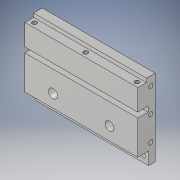
# Autodesk Inventor part: Стенка толстая
Saved by Autodesk Inventor 2019 (Build 230136000, 136)
## iProperties
Company: КВ33
Created: 2021-03-13
Part Number: Стенка толстая
Material: Типовые
Document SubType Name: Modeling
Designer: Петров Иван
Density: 1 g/cm^3
Appearance: Aluminum - Polished
Author: Петров Иван
Autodesk Inventor part; units mm, degrees
ref_plane "YZ Plane" through (0, 0, 0) normal (1, 0, 0) x (0, 1, 0)
ref_plane "XZ Plane" through (0, 0, 0) normal (0, 1, 0) x (-1, 0, 0)
ref_plane "XY Plane" through (0, 0, 0) normal (0, 0, 1) x (1, 0, 0)
sketch "Sketch1" plane through (0, 0, 0) normal (0, 0, 1) x (1, 0, 0)
  line L0 (50.1275, 12.4589) -> (-37.8725, 12.4589) projected
  line L1 (50.1275, 12.4589) -> (-37.8725, 12.4589)
  line L2 (-37.8725, 12.4589) -> (-37.8725, 62.4589)
  line L3 (-37.8725, 62.4589) -> (50.1275, 62.4589)
  line L4 (50.1275, 62.4589) -> (50.1275, 12.4589)
  circle A0 centre (-33.8725, 7.4589) radius 1.75 projected
  circle A1 centre (-13.8725, 7.4589) radius 1.75 projected
  circle A2 centre (6.1275, 7.4589) radius 1.75 projected
  circle A3 centre (26.1275, 7.4589) radius 1.75 projected
  circle A4 centre (46.1275, 7.4589) radius 1.75 projected
  line L5 (-37.8725, 2.4589) -> (50.1275, 2.4589) projected
  line L6 (-37.8725, 2.4589) -> (-37.8725, 12.4589) projected
  line L7 (50.1275, 12.4589) -> (-37.8725, 12.4589) projected
  line L8 (50.1275, 2.4589) -> (50.1275, 12.4589) projected
  line L9 (50.1275, -7.5411) -> (-37.8725, -7.5411) projected
  line L10 (-37.8725, -7.5411) -> (-37.8725, 2.4589) projected
  line L11 (50.1275, 2.4589) -> (-37.8725, 2.4589) projected
  line L12 (50.1275, -7.5411) -> (50.1275, 2.4589) projected
  dimension "d0" = 50
  dimension "d1" = 88
  constraints: 8 end point, 2 parallel, 1 horizontal, 1 perpendicular
  measures "d0" distance of L1.end L2.end
  measures "d1" distance of L2.end L3.end
ref_plane "Work Plane1" through (-40.3725, -19.5411, 5) normal (0, 0, -1) x (0, 1, 0)
extrude "Extrusion1" add sketch "Sketch1" along normal up to surface (5 mm away) contours L8 L5 L6 L0
sketch "Sketch2" plane through (0, 0, 0) normal (0, 0, -1) x (-1, 0, 0)
  line L0 (37.8725, -7.5411) -> (-50.1275, -7.5411)
  line L1 (-50.1275, -7.5411) -> (-50.1275, 2.4589)
  line L2 (37.8725, 2.4589) -> (-50.1275, 2.4589)
  line L3 (37.8725, -7.5411) -> (37.8725, 2.4589)
  circle A0 centre (-46.1275, 7.4589) radius 1.75
  circle A1 centre (-26.1275, 7.4589) radius 1.75
  circle A2 centre (-6.1275, 7.4589) radius 1.75
  circle A3 centre (13.8725, 7.4589) radius 1.75
  circle A4 centre (33.8725, 7.4589) radius 1.75
  line L4 (-50.1275, 2.4589) -> (37.8725, 2.4589)
  line L5 (-50.1275, 2.4589) -> (-50.1275, 12.4589)
  line L6 (37.8725, 12.4589) -> (-50.1275, 12.4589)
  line L7 (37.8725, 2.4589) -> (37.8725, 12.4589)
  line L8 (37.8725, 12.4589) -> (-50.1275, 12.4589)
  line L9 (-50.1275, 12.4589) -> (-50.1275, 62.4589)
  line L10 (-50.1275, 62.4589) -> (37.8725, 62.4589)
  line L11 (37.8725, 62.4589) -> (37.8725, 12.4589)
  line L12 (-50.1275, 2.4589) -> (-50.1275, 12.4589) projected
  point P0 (0, 0)
  point P1 (-12.255, 0)
  dimension "d4" = 50
  dimension "d5" = 88
  constraints: 24 end point, 5 centre point, 2 parallel, 1 horizontal, 1 perpendicular
  measures "d4" distance of L8.end L9.end
  measures "d5" distance of L9.end L10.end
ref_plane "Work Plane2" through (-22.976, -19.3597, 13.5507) normal (0, 0, 1) x (1, 0, 0)
extrude "Extrusion2" add sketch "Sketch2" against normal up to surface (13.5507 mm away) contours L6 L9 L10 L11
sketch "Sketch6" plane through (-37.8725, 62.4589, 0) normal (0, 1, 0) x (1, 0, 0)
  line L0 (88, -13.5507) -> (0, -13.5507) projected
  line L1 (88, 0) -> (88, -13.5507) projected
  line L2 (0, -13.5507) -> (88, -13.5507)
  line L3 (88, -13.5507) -> (88, -6.7754)
  line L4 (88, -6.7754) -> (0, -6.7754)
  line L5 (0, -6.7754) -> (0, -13.5507)
  point P0 (37.8725, 0)
  constraints: 8 end point, 2 parallel, 1 horizontal, 1 midpoint, 1 perpendicular
extrude "Extrusion6" cut sketch "Sketch6" against normal blind 3
sketch "Sketch7" plane through (50.1275, 2.4589, 5) normal (1, 0, 0) x (0, 0, -1)
  circle A0 centre (1.6123, 52.8914) radius 1.75
  line L0 (5, 0) -> (5, 60) projected
  line L1 (-1.7754, 60) -> (-1.7754, 57) projected
  point P0 (5, -2.4589)
  dimension "d30" = 3.5
  dimension "d31" = 3.3877
  dimension "d32" = 6.7754
  constraints: 1 centre point
  measures "d30" diameter of A0
  measures "d31" distance from line of L0 A0.centre
  measures "d32" distance between parallel lines of L0 L1
hole "Hole1" at (50.1275, 55.3502, 3.3877) direction (-1, 0, 0) diameter 3.5 depth 10 tip angle 120
thread "Thread2" size "M3.5x0.6" class "6H" standard "ANSI Metric M Profile" full length
pattern_linear "Rectangular Pattern2" count 3 spacing 19 along (0, -1, 0) of "Hole1"
ref_plane "Work Plane5" through (6.1275, 62.4589, 0) normal (1, 0, 0) x (0, 0, -1)
mirror "Mirror2" about plane through (6.1275, 62.4589, 0) normal (1, 0, 0) of "Hole1", "Rectangular Pattern2"
sketch "Sketch8" plane through (-37.8725, 59.4589, 0) normal (0, 1, 0) x (1, 0, 0)
  circle A0 centre (84, -10.0507) radius 1.75
  line L0 (88, -13.5507) -> (0, -13.5507) projected
  line L1 (88, -6.7754) -> (88, -13.5507) projected
  point P0 (37.8725, 0)
  dimension "d45" = 3.5
  dimension "d46" = 3.5
  dimension "d47" = 4
  constraints: 1 centre point
  measures "d45" diameter of A0
  measures "d46" distance from line of L0 A0.centre
  measures "d47" distance from line of L1 A0.centre
hole "Hole2" at (46.1275, 59.4589, 10.0507) direction (0, -1, 0) diameter 3.5 depth 8 tip angle 120
thread "Thread3" size "M3.5x0.6" class "6H" standard "ANSI Metric M Profile" full length
pattern_linear "Rectangular Pattern3" count 3 spacing 40 along (-1, 0, 0) of "Hole2"
sketch "Sketch9" plane through (0, 0, 0) normal (0, 0, -1) x (-1, 0, 0)
  line L0 (18.226, -7.5411) -> (18.226, 11.4589) projected
  line L1 (4.4437, -7.5411) -> (4.4437, -52.4226) projected
  line L2 (37.8725, 2.4589) -> (-50.1275, 2.4589) projected
  line L3 (37.8725, 62.4589) -> (-50.1275, 62.4589) projected
  circle A0 centre (15.8725, 22.4589) radius 9.5
  line L4 (37.8725, 2.4589) -> (-50.1275, 2.4589) projected
  point P0 (0, 0)
  point P1 (15.8725, 2.4589)
  point P2 (-6.1275, 62.4589)
  dimension "d60" = 19
  dimension "d69" = 20
  dimension "d74" = 22
  constraints: 1 centre point, 1 midpoint, 1 point on line, 1 vertical alignment
  measures "d60" diameter of A0
  measures "d69" distance of A0.centre point (15.872, 2.459)
  measures "d74" horizontal distance of point (15.872, 2.459) point (-6.128, 62.459)
extrude "Extrusion7" cut sketch "Sketch9" against normal blind 6
sketch "Sketch10" plane through (-15.8725, 22.4589, 6) normal (0, 0, -1) x (-1, 0, 0)
  circle A0 centre (0, 0) radius 3.5
  point P0 (-15.8725, -22.4589)
  dimension "d63" = 7
  constraints: 1 centre point
  measures "d63" diameter of A0
extrude "Extrusion8" cut sketch "Sketch10" against normal blind 15.25
ref_plane "Work Plane6" through (6.1275, 62.4589, 0) normal (1, 0, 0) x (0, 0, -1)
mirror "Mirror3" about plane through (6.1275, 62.4589, 0) normal (1, 0, 0) of "Extrusion7", "Extrusion8"
chamfer "Chamfer1" distance 0.5 angle 45 2 edges at (18.6275, 22.4589, 0) (-6.3725, 22.4589, 0)
sketch "Sketch11" plane through (50.1275, 2.4589, 5) normal (1, 0, 0) x (0, 0, -1)
  line L0 (-1, 10.5) -> (-1, 29.5) projected
  line L1 (4.5, 29.5) -> (4.5, 10.5) projected
  circle A0 centre (1.6123, 14.8914) radius 1.75 projected
  circle A1 centre (1.6123, 33.8914) radius 1.75 projected
  circle A2 centre (1.6123, 52.8914) radius 1.75 projected
  line L2 (-1.7754, 57) -> (-8.5507, 57) projected
  line L3 (-8.5507, 57) -> (-8.5507, 10) projected
  line L4 (0, 10) -> (-8.5507, 10) projected
  line L5 (0, 0) -> (0, 10) projected
  line L6 (5, 0) -> (0, 0) projected
  line L7 (5, 0) -> (5, 60) projected
  line L8 (5, 60) -> (-1.7754, 60) projected
  line L9 (-1.7754, 60) -> (-1.7754, 57) projected
  line L10 (-8.5507, 10) -> (-8.5507, 57) projected
  line L11 (-8.5507, 40.4435) -> (-0.5507, 40.4435)
  line L12 (-0.5507, 40.4435) -> (-0.5507, 36.4435)
  line L13 (-0.5507, 36.4435) -> (-8.5507, 36.4435)
  line L14 (-8.5507, 36.4435) -> (-8.5507, 40.4435)
  point P0 (5, -2.4589)
  dimension "d70" = 4
  dimension "d73" = 8
  constraints: 8 end point, 2 parallel, 1 horizontal, 1 perpendicular, 1 point on line
  measures "d70" distance between parallel lines of L13 L11
  measures "d73" distance between parallel lines of L3 L12
extrude "Extrusion9" cut sketch "Sketch11" against normal blind 102.5 contours L11 L12 L13 L3
equation "\"d31\" = 0.5 * d32"
body "Solid1"
